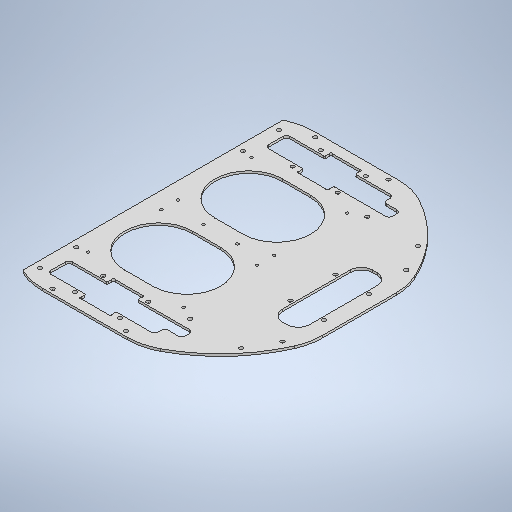
# Autodesk Inventor part: T2.0_frame-base1
Saved by Autodesk Inventor 2025 (Build 290162000, 162)
## iProperties
Created: 2024-06-26
Part Number: T2.0_frame-base1
Material: 一般
Document SubType Name: Sheet Metal
Designer: 8326d
Density: 1 g/cm^3
Sheet Metal Rule: Default_mm
Appearance: 既定
Author: 8326d
Autodesk Inventor part; units mm, degrees
ref_plane "YZ Plane" through (0, 0, 0) normal (1, 0, 0) x (0, 1, 0)
ref_plane "XZ Plane" through (0, 0, 0) normal (0, 1, 0) x (-1, 0, 0)
ref_plane "XY Plane" through (0, 0, 0) normal (0, 0, 1) x (1, 0, 0)
sketch "スケッチ1" plane through (0, 0, 0) normal (0, 1, 0) x (-1, 0, 0)
  circle A0 centre (0, 0) radius 130
  dimension "d0" = 260
  measures "d0" diameter of A0
extrude "プレート1" add sketch "スケッチ1" along normal blind 2
sketch "スケッチ2" plane through (0, 2, 0) normal (0, 1, 0) x (1, 0, 0)
  line L0 (85, -40) -> (109, -40)
  line L1 (109, -40) -> (109, 40)
  line L2 (109, 40) -> (85, 40)
  line L3 (85, 40) -> (85, -40)
  line L4 (85, -40) -> (109, 40) construction
  line L5 (109, -40) -> (85, 40) construction
  point P0 (0, 0)
  point P1 (97, 0)
  dimension "d2" = 24
  dimension "d3" = 85
  dimension "d6" = 80
  constraints: 12 end point, 2 midpoint, 2 parallel, 1 horizontal, 1 horizontal alignment, 1 perpendicular
  measures "d2" distance of L1.end L2.end
  measures "d3" distance from line of point (0, 0) L3
  measures "d6" distance of L0.end L1.end
extrude "押し出し1" cut sketch "スケッチ2" against normal through all
fillet "フィレット1" radius 10 4 edges at (109, 1, 40) (85, 1, 40) (85, 1, -40) (109, 1, -40)
sketch "スケッチ3" plane through (0, 2, 0) normal (0, 1, 0) x (1, 0, 0)
  line L0 (85, -30) -> (85, 30) projected
  line L1 (109, 30) -> (109, -30) projected
  line L2 (95, 40) -> (99, 40) projected
  line L3 (99, -40) -> (95, -40) projected
  line L4 (82, -20) -> (112, -20) construction
  line L5 (112, -20) -> (112, 20) construction
  line L6 (112, 20) -> (82, 20) construction
  line L7 (82, 20) -> (82, -20) construction
  line L8 (82, -20) -> (112, 20) construction
  line L9 (112, -20) -> (82, 20) construction
  point P0 (0, 0)
  point P1 (97, 0)
  point P2 (97, 40)
  point P3 (109, 0)
  dimension "d8" = 30
  dimension "d9" = 40
  constraints: 12 end point, 4 midpoint, 2 parallel, 1 horizontal, 1 horizontal alignment, 1 perpendicular, 1 vertical alignment
  measures "d8" distance of L6.end L5.end
  measures "d9" distance of L5.end L4.end
hole "穴1" at (82, 2, 20) at (112, 2, 20) at (112, 2, -20) at (82, 2, -20) direction (0, -1, 0) diameter 3.5 depth 2 tip angle 118
sketch "スケッチ4" plane through (0, 2, 0) normal (0, 1, 0) x (1, 0, 0)
  circle A0 centre (0, 0) radius 130 projected
  line L0 (-106.1838, 75) -> (-60, 40)
  line L1 (-60, 40) -> (-60, -40)
  line L2 (-60, -40) -> (-106.1838, -75)
  point P0 (-60, 0)
  dimension "d17" = 40
  dimension "d18" = 75
  dimension "d19" = 60
  constraints: 6 end point, 2 point on circle, 1 horizontal alignment, 1 midpoint, 1 vertical, 1 vertical alignment
  measures "d17" vertical distance of L1.end point (0, 0)
  measures "d18" vertical distance of point (0, 0) L0.start
  measures "d19" distance from line of point (0, 0) L1
extrude "押し出し2" cut sketch "スケッチ4" against normal through all contours L0 L1 L2 A0 picked at (-83.3333, 0)
sketch "スケッチ5" plane through (0, 2, 0) normal (0, 1, 0) x (1, 0, 0)
  line L0 (-47.5, 87) -> (47.5, 87)
  line L1 (47.5, 87) -> (47.5, 106)
  line L2 (47.5, 106) -> (-47.5, 106)
  line L3 (-47.5, 106) -> (-47.5, 87)
  line L4 (-47.5, 87) -> (47.5, 106) construction
  line L5 (47.5, 87) -> (-47.5, 106) construction
  line L6 (-13.5, 81.5) -> (13.5, 81.5)
  line L7 (13.5, 81.5) -> (13.5, 87)
  line L8 (13.5, 87) -> (-13.5, 87)
  line L9 (-13.5, 87) -> (-13.5, 81.5)
  line L10 (-13.5, 81.5) -> (13.5, 87) construction
  line L11 (13.5, 81.5) -> (-13.5, 87) construction
  line L12 (-13.5, 81.5) -> (-12.7575, 82.2425) construction
  line L13 (-13.5, 81.5) -> (-12.45, 81.5) construction
  line L14 (13.5, 81.5) -> (12.7575, 82.2425) construction
  line L15 (13.5, 81.5) -> (14.55, 81.5) construction
  circle A0 centre (12.7575, 82.2425) radius 1.05
  circle A1 centre (-12.7575, 82.2425) radius 1.05
  line L16 (47.5, 87) -> (62.5, 87)
  line L17 (62.5, 87) -> (62.5, 97)
  line L18 (62.5, 97) -> (47.5, 97)
  line L19 (47.5, 97) -> (47.5, 87)
  line L20 (-13.5, 111.5) -> (13.5, 111.5)
  line L21 (13.5, 111.5) -> (13.5, 106)
  line L22 (13.5, 106) -> (-13.5, 106)
  line L23 (-13.5, 106) -> (-13.5, 111.5)
  line L24 (-13.5, 111.5) -> (13.5, 106) construction
  line L25 (13.5, 111.5) -> (-13.5, 106) construction
  line L26 (-13.5, 111.5) -> (-12.7575, 110.7575) construction
  line L27 (-13.5, 111.5) -> (-12.45, 111.5) construction
  line L28 (13.5, 111.5) -> (12.7575, 110.7575) construction
  line L29 (13.5, 111.5) -> (14.55, 111.5) construction
  circle A2 centre (-12.7575, 110.7575) radius 1.05
  circle A3 centre (12.7575, 110.7575) radius 1.05
  point P0 (0, 0)
  point P1 (0, 96.5)
  point P2 (0, 84.25)
  point P3 (-13.5, 82.9849)
  point P4 (-12.0151, 81.5)
  point P5 (12.0151, 81.5)
  point P6 (13.5, 82.9849)
  point P7 (47.5, 97)
  point P8 (0, 108.75)
  point P9 (-13.5, 110.0151)
  point P10 (13.5, 110.0151)
  point P11 (12.0151, 111.5)
  point P12 (-12.0151, 111.5)
  dimension "d22" = 19
  dimension "d23" = 95
  dimension "d24" = 87
  dimension "d25" = 5.5
  dimension "d26" = 27
  dimension "d27" = 1.05
  dimension "d28" = 45
  dimension "d29" = 1.05
  dimension "d30" = 135
  dimension "d44" = 10
  dimension "d45" = 15
  dimension "d46" = 5.5
  dimension "d47" = 1.05
  dimension "d48" = 45
  dimension "d49" = 1.05
  dimension "d50" = 135
  constraints: 60 end point, 8 horizontal, 8 parallel, 6 midpoint, 4 coincident, 4 equal length, 4 perpendicular, 4 vertical alignment, 2 point on line, 12 other
  measures "d22" distance of L0.end L1.end
  measures "d23" distance of L1.end L2.end
  measures "d24" distance from line of point (0, 0) L0
  measures "d25" distance of L6.end L7.end
  measures "d26" distance of L6.start L6.end
  measures "d27" distance of L6.start L12.end
  measures "d28" angle of L13 L12
  measures "d29" distance of L6.end L14.end
  measures "d30" angle of L15 L14
  measures "d44" distance of L16.end L17.end
  measures "d45" distance of L17.end L18.end
  measures "d46" distance between parallel lines of L2 L20
  measures "d47" distance of L20.start L26.end
  measures "d48" angle of L26 L27
  measures "d49" distance of L20.end L28.end
  measures "d50" angle of L28 L29
extrude "押し出し3" cut sketch "スケッチ5" against normal through all
sketch "スケッチ6" plane through (0, 2, 0) normal (0, 1, 0) x (1, 0, 0)
  line L0 (-20, 84) -> (20, 84) construction
  line L1 (-20, 84) -> (20, 84) construction
  line L2 (12.0151, 81.5) -> (-12.0151, 81.5) construction
  line L3 (-20, 109) -> (20, 109) construction
  line L4 (13.5, 106) -> (47.5, 106) construction
  line L5 (-20, 109) -> (20, 109) construction
  line L6 (-12.0151, 111.5) -> (12.0151, 111.5) construction
  point P0 (0, 0)
  point P1 (0, 84)
  point P2 (0, 109)
  point P3 (0, 84)
  dimension "d33" = 40
  dimension "d34" = 0
  dimension "d35" = 2.5
  dimension "d51" = 40
  dimension "d52" = 0
  dimension "d53" = 2.5
  constraints: 8 end point, 3 horizontal, 3 midpoint, 2 collinear, 2 vertical alignment, 1 parallel
  measures "d33" distance of L0.start L0.end
  measures "d34" distance between parallel lines of L0 L1
  measures "d35" distance between parallel lines of L0 L2
  measures "d51" distance of L3.start L3.end
  measures "d52" distance between parallel lines of L3 L5
  measures "d53" distance between parallel lines of L6 L3
hole "穴2" at (20, 2, -84) at (-20, 2, -84) at (-20, 2, -109) at (20, 2, -109) direction (0, -1, 0) diameter 3.5 depth 2 tip angle 118
fillet "フィレット2" radius 1 4 edges at (-13.5, 1, -87) (13.5, 1, -87) (-13.5, 1, -106) (13.5, 1, -106)
fillet "フィレット3" radius 3 6 edges at (-47.5, 1, -87) (-47.5, 1, -106) (47.5, 1, -106) (47.5, 1, -97) (62.5, 1, -97) (62.5, 1, -87)
mirror "ミラー1" about plane through (0, 0, 0) normal (0, 0, 1) of "穴2", "押し出し3", "フィレット2", "フィレット3"
sketch "スケッチ7" plane through (0, 2, 0) normal (0, 1, 0) x (1, 0, 0)
  arc A0 (-106.1838, -75) -> (-106.1838, 75) centre (0, 0) ccw projected
  line L0 (-48.7827, 120.5) -> (48.7827, 120.5)
  line L1 (-48.7827, -120.5) -> (48.7827, -120.5)
  line L2 (123, -42.0833) -> (123, 42.0833)
  line L3 (-12.0151, 111.5) -> (12.0151, 111.5) projected
  circle A1 centre (112, 20) radius 1.75 projected
  line L4 (12.0151, -111.5) -> (-12.0151, -111.5) projected
  dimension "d55" = 9
  dimension "d56" = 11
  dimension "d57" = 9
  constraints: 6 end point, 6 point on circle, 1 horizontal, 1 parallel, 1 perpendicular
  measures "d55" distance between parallel lines of L3 L0
  measures "d56" distance from line of A1.centre L2
  measures "d57" distance between parallel lines of L1 L4
extrude "押し出し4" cut sketch "スケッチ7" against normal through all contours L1 A0 | L2 A0 | L0 A0
fillet "フィレット4" radius 50 6 edges at (48.7827, 1, 120.5) (-48.7827, 1, 120.5) (123, 1, 42.0833) (123, 1, -42.0833) (48.7827, 1, -120.5) (-48.7827, 1, -120.5)
sketch "スケッチ8" plane through (0, 0, 0) normal (0, -1, 0) x (1, 0, 0)
  arc A0 (97.4046, 79.5902) -> (95.9996, 79.4659) centre (96.7931, 78.5) ccw projected
  arc A1 (52.5865, 79.4659) -> (51.1816, 79.5902) centre (51.7931, 78.5) ccw projected
  point P0 (0, 0)
hole "穴3" at (96.7931, 0, 78.5) at (51.7931, 0, 78.5) direction (0, 1, 0) diameter 3.5 depth 2 tip angle 118
sketch "スケッチ10" plane through (0, 2, 0) normal (0, 1, 0) x (1, 0, 0)
  line L0 (-32.5, -116.5) -> (32.5, -116.5) construction
  line L1 (-32.5, -116.5) -> (32.5, -116.5) construction
  line L2 (-37.812, -120.5) -> (37.812, -120.5) construction
  point P0 (0, 0)
  point P1 (0, -116.5)
  dimension "d78" = 65
  dimension "d79" = 0
  dimension "d80" = 4
  constraints: 4 end point, 2 horizontal, 1 collinear, 1 midpoint, 1 vertical alignment
  measures "d78" distance of L0.start L0.end
  measures "d79" distance between parallel lines of L0 L1
  measures "d80" distance between parallel lines of L2 L0
hole "穴5" at (32.5, 2, 116.5) at (-32.5, 2, 116.5) direction (0, -1, 0) diameter 3.5 end through all
mirror "ミラー2" about plane through (0, 0, 0) normal (0, 0, 1) of "穴3", "穴5"
sketch "スケッチ9" plane through (0, 2, 0) normal (0, 1, 0) x (1, 0, 0)
  line L0 (110, -55) -> (110, 55) construction
  line L1 (109, 30) -> (109, -30) construction
  line L2 (110, -55) -> (220, -55) construction
  point P0 (0, 0)
  point P1 (110, 0)
  dimension "d68" = 110
  dimension "d69" = 90
  dimension "d70" = 110
  constraints: 4 end point, 1 horizontal, 1 horizontal alignment, 1 midpoint, 1 parallel, 1 perpendicular
  measures "d68" distance of L0.start L0.end
  measures "d69" angle of L2 L0
  measures "d70" distance from line of point (0, 0) L0
hole "穴4" at (110, 2, 55) at (110, 2, -55) direction (0, -1, 0) diameter 3.5 depth 2 tip angle 118
sketch "スケッチ11" plane through (0, 2, 0) normal (0, 1, 0) x (1, 0, 0)
  line L0 (-45, 7.5) -> (40, 7.5) construction
  line L1 (40, 7.5) -> (40, 72.5) construction
  line L2 (40, 72.5) -> (-45, 72.5) construction
  line L3 (-45, 72.5) -> (-45, 7.5) construction
  line L4 (-45, 7.5) -> (40, 72.5) construction
  line L5 (40, 7.5) -> (-45, 72.5) construction
  line L6 (-60, 40) -> (-60, -40) construction
  point P0 (0, 0)
  point P1 (-2.5, 40)
  dimension "d88" = 85
  dimension "d89" = 65
  dimension "d90" = 7.5
  dimension "d91" = 15
  constraints: 12 end point, 2 midpoint, 2 parallel, 1 horizontal, 1 perpendicular
  measures "d88" distance of L2.end L1.end
  measures "d89" distance of L1.end L0.end
  measures "d90" distance from line of point (0, 0) L0
  measures "d91" distance between parallel lines of L6 L3
hole "穴6" at (-45, 2, -7.5) at (40, 2, -7.5) at (40, 2, -72.5) at (-45, 2, -72.5) direction (0, -1, 0) diameter 2.5 end through all
sketch "スケッチ12" plane through (0, 2, 0) normal (0, 1, 0) x (1, 0, 0)
  line L0 (-15, 40) -> (10, 40) construction
  line L1 (-15, 10) -> (10, 10)
  line L2 (10, 70) -> (-15, 70)
  arc A0 (-15, 70) -> (-15, 10) centre (-15, 40) ccw
  arc A1 (10, 10) -> (10, 70) centre (10, 40) ccw
  circle A2 centre (-45, 72.5) radius 1.25 projected
  circle A3 centre (-45, 7.5) radius 1.25 projected
  point P0 (0, 0)
  point P1 (-2.5, 40)
  dimension "d99" = 25
  dimension "d100" = 30
  dimension "d101" = 42.5
  dimension "d102" = 32.5
  constraints: 8 end point, 4 point on circle, 4 tangent, 2 centre point, 1 horizontal, 1 midpoint, 1 parallel
  measures "d99" distance of L0.start L0.end
  measures "d100" radius of A1
  measures "d101" horizontal distance of A2.centre point (-2.5, 40)
  measures "d102" vertical distance of A3.centre point (-2.5, 40)
extrude "押し出し5" cut sketch "スケッチ12" against normal through all contours A0 L2 A1 L1
mirror "ミラー3" about plane through (0, 0, 0) normal (0, 0, 1) of "穴6", "押し出し5"
sketch "スケッチ13" plane through (0, 2, 0) normal (0, 1, 0) x (1, 0, 0)
  line L0 (-15, 0) -> (15, 0) construction
  line L1 (-15, 0) -> (15, 0) construction
  point P0 (0, 0)
  point P1 (0, 0)
  dimension "d105" = 30
  dimension "d106" = 0
  constraints: 4 end point, 2 horizontal, 1 coincident, 1 collinear, 1 midpoint
  measures "d105" distance of L0.start L0.end
  measures "d106" distance between parallel lines of L0 L1
hole "穴7" at (-15, 2, 0) at (15, 2, 0) direction (0, -1, 0) diameter 2.5 end through all
sketch "スケッチ14" plane through (0, 2, 0) normal (0, 1, 0) x (1, 0, 0)
  line L0 (-106.1838, 75) -> (-60, 40) projected
  arc A0 (-61.4446, 114.5625) -> (-106.1838, 75) centre (0, 0) ccw projected
  line L1 (-60, -40) -> (-106.1838, -75) projected
  arc A1 (-106.1838, -75) -> (-61.4446, -114.5625) centre (0, 0) ccw projected
  line L2 (-102.4695, 80) -> (-102.4695, -80)
  line L3 (-102.4695, 80) -> (57.5305, 80) construction
  point P0 (-102.4695, 72.1852)
  point P1 (-102.4695, -72.1852)
  dimension "d114" = 160
  dimension "d115" = 90
  constraints: 4 end point, 2 point on circle, 1 horizontal, 1 perpendicular, 1 vertical
  measures "d114" distance of L2.start L2.end
  measures "d115" angle of L2 L3
extrude "押し出し6" cut sketch "スケッチ14" against normal through all
sketch "スケッチ15" plane through (0, 2, 0) normal (0, 1, 0) x (1, 0, 0)
  line L0 (-92.9695, -76.5) -> (-82.9695, -76.5) construction
  line L1 (-82.9695, -76.5) -> (-82.9695, 76.5) construction
  line L2 (-82.9695, 76.5) -> (-92.9695, 76.5) construction
  line L3 (-92.9695, 76.5) -> (-92.9695, -76.5) construction
  line L4 (-92.9695, -76.5) -> (-82.9695, 76.5) construction
  line L5 (-82.9695, -76.5) -> (-92.9695, 76.5) construction
  line L6 (-102.4695, 80) -> (-102.4695, 72.1852) construction
  point P0 (0, 0)
  point P1 (-87.9695, 0)
  dimension "d118" = 10
  dimension "d119" = 153
  dimension "d120" = 9.5
  constraints: 12 end point, 4 coincident, 2 midpoint, 2 parallel, 1 horizontal, 1 horizontal alignment, 1 perpendicular
  measures "d118" distance of L2.end L1.end
  measures "d119" distance of L1.end L0.end
  measures "d120" distance between parallel lines of L6 L3
hole "穴8" at (-92.9695, 2, -76.5) at (-82.9695, 2, -76.5) at (-82.9695, 2, 76.5) at (-92.9695, 2, 76.5) direction (0, -1, 0) diameter 3.5 end through all
sketch "スケッチ16" plane through (0, 0, 0) normal (0, -1, 0) x (1, 0, 0)
  circle A0 centre (-94.9691, 83.565) radius 1.75 projected
  circle A1 centre (-82.3072, 96.0613) radius 1.75 projected
  circle A2 centre (-94.9691, 83.565) radius 1.75 projected
  point P0 (0, 0)
hole "穴9" at (-94.9691, 0, 83.565) at (-82.3072, 0, 96.0613) direction (0, 1, 0) diameter 3.5 depth 2
mirror "ミラー4" about plane through (0, 0, 0) normal (0, 0, 1) of "穴9"
fillet "フィレット5" radius 2 6 edges at (-102.4695, 1, -72.1852) (-102.4695, 1, -80) (-60, 1, -40) (-60, 1, 40) (-102.4695, 1, 80) (-102.4695, 1, 72.1852)
sketch "スケッチ20" plane through (0, 2, 0) normal (0, 1, 0) x (1, 0, 0)
  line L0 (-60, 39.0062) -> (-60, -39.0062) projected
  arc A0 (-61.4446, 114.5625) -> (-102.0393, 80.548) centre (0, 0) ccw projected
  arc A1 (-102.0393, -80.548) -> (-61.4446, -114.5625) centre (0, 0) ccw projected
  arc A2 (-61.4446, -114.5625) -> (-37.812, -120.5) centre (-37.812, -70.5) ccw projected
  arc A3 (-37.812, 120.5) -> (-61.4446, 114.5625) centre (-37.812, 70.5) ccw projected
  line L1 (-60, 39.0062) -> (-60, 115.3073) construction
  line L2 (-60, -39.0062) -> (-60, -115.3073) construction
  line L3 (-66, 74) -> (-54, 74) construction
  line L4 (-54, 74) -> (-54, 106) construction
  line L5 (-54, 106) -> (-66, 106) construction
  line L6 (-66, 106) -> (-66, 74) construction
  line L7 (-66, 74) -> (-54, 106) construction
  line L8 (-54, 74) -> (-66, 106) construction
  line L9 (-66, -106) -> (-54, -106) construction
  line L10 (-54, -106) -> (-54, -74) construction
  line L11 (-54, -74) -> (-66, -74) construction
  line L12 (-66, -74) -> (-66, -106) construction
  line L13 (-66, -106) -> (-54, -74) construction
  line L14 (-54, -106) -> (-66, -74) construction
  point P0 (-60, 90)
  point P1 (-60, -90)
  dimension "d155" = 12
  dimension "d156" = 32
  dimension "d157" = 12
  dimension "d158" = 32
  dimension "d169" = 90
  dimension "d170" = 90
  constraints: 28 end point, 4 midpoint, 4 parallel, 2 collinear, 2 horizontal, 2 perpendicular, 2 point on circle, 2 point on line
  measures "d155" distance of L5.end L4.end
  measures "d156" distance of L4.end L3.end
  measures "d157" distance of L11.end L10.end
  measures "d158" distance of L10.end L9.end
  measures "d169" vertical distance of point (0, 0) point (-60, 90)
  measures "d170" vertical distance of point (0, 0) point (-60, -90)
hole "穴10" at (-54, 2, -74) at (-66, 2, -74) at (-66, 2, -106) at (-54, 2, -106) at (-66, 2, 74) at (-54, 2, 74) at (-54, 2, 106) at (-66, 2, 106) direction (0, -1, 0) diameter 3.5 depth 2
sketch "スケッチ21" plane through (0, 2, 0) normal (0, 1, 0) x (1, 0, 0)
  line L0 (-60, 39.0062) -> (-60, -39.0062) projected
  arc A0 (-61.4446, -114.5625) -> (-37.812, -120.5) centre (-37.812, -70.5) ccw projected
  arc A1 (-37.812, 120.5) -> (-61.4446, 114.5625) centre (-37.812, 70.5) ccw projected
  arc A2 (-61.4446, 114.5625) -> (-102.0393, 80.548) centre (0, 0) ccw projected
  arc A3 (-102.0393, -80.548) -> (-61.4446, -114.5625) centre (0, 0) ccw projected
  line L1 (-60, 39.0062) -> (-60, 115.3073)
  line L2 (-60.792, -40.6002) -> (-101.6775, -71.5849) projected
  line L3 (-60, -39.0062) -> (-60, -118.5898)
  line L4 (-102.4695, -73.1789) -> (-102.4695, -79.3088) projected
  arc A4 (-101.6775, -71.5849) -> (-102.4695, -73.1789) centre (-100.4695, -73.1789) ccw projected
  arc A5 (-102.4695, -79.3088) -> (-102.0393, -80.548) centre (-100.4695, -79.3088) ccw projected
  line L5 (-101.6775, 71.5849) -> (-60.792, 40.6002) projected
  line L6 (-102.4695, 79.3088) -> (-102.4695, 73.1789) projected
  arc A6 (-102.4695, 73.1789) -> (-101.6775, 71.5849) centre (-100.4695, 73.1789) ccw projected
  arc A7 (-102.0393, 80.548) -> (-102.4695, 79.3088) centre (-100.4695, 79.3088) ccw projected
  arc A8 (-60, 39.0062) -> (-60.792, 40.6002) centre (-62, 39.0062) ccw projected
  arc A9 (-60.792, -40.6002) -> (-60, -39.0062) centre (-62, -39.0062) ccw projected
  point P0 (-60.0015, 39.0827)
  point P1 (-60, -115.3073)
  constraints: 4 end point, 2 collinear, 1 point on circle
extrude "押し出し10" cut sketch "スケッチ21" against normal through all
fillet "フィレット6" radius 1 2 edges at (-60, 1, 115.3073) (-60, 1, -115.3073)
equation "\"d15\" = Thickness"
equation "\"d46\" = d25"
equation "\"d53\" = d35"
equation "\"d41\" = Thickness"
equation "\"d57\" = d55"
equation "\"d66\" = Thickness"
equation "\"d86\" = Thickness"
equation "\"d76\" = Thickness"
equation "\"d1\" = Thickness"
equation "\"BendRadius\" = Thickness"
equation "\"BendReliefWidth\" = Thickness"
equation "\"BendReliefDepth\" = 0.5 * Thickness"
equation "\"CornerReliefSize\" = 4 * Thickness"
equation "\"MinimumRemnant\" = 2 * Thickness"
equation "\"TransitionRadius\" = BendRadius"
equation "\"JacobiRadiusSize\" = BendRadius"
equation "\"GapSize\" = Thickness"
equation "\"Thickness\" = 2"
